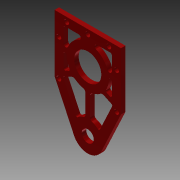
# Autodesk Inventor part: Swerve Wheel + Carriage Outline V1
Saved by Autodesk Inventor 2013 (Build 170138000, 138)
## iProperties
Created: 2013-04-01
Part Number: Swerve Wheel + Carriage Outline V1
Material: Generic
Document SubType Name: Sheet Metal
Designer: mvarma
Density: 1 g/cm^3
Sheet Metal Rule: Default
Author: mvarma
Autodesk Inventor part; units mm, degrees
ref_plane "YZ Plane" through (0, 0, 0) normal (1, 0, 0) x (0, 1, 0)
ref_plane "XZ Plane" through (0, 0, 0) normal (0, 1, 0) x (-1, 0, 0)
ref_plane "XY Plane" through (0, 0, 0) normal (0, 0, 1) x (1, 0, 0)
sketch "Sketch1" plane through (0, 0, 0) normal (0, 0, 1) x (1, 0, 0)
  circle A0 centre (0, 0) radius 38.1 construction
  circle A1 centre (0, 0) radius 41.275 construction
  line L0 (-7.332348, 0) -> (-3.666174, 6.35) construction
  line L1 (-3.666174, 6.35) -> (3.666174, 6.35) construction
  line L2 (3.666174, 6.35) -> (7.332348, 0) construction
  line L3 (7.332348, 0) -> (3.666174, -6.35) construction
  line L4 (3.666174, -6.35) -> (-3.666174, -6.35) construction
  line L5 (-3.666174, -6.35) -> (-7.332348, 0) construction
  circle A2 centre (0, 0) radius 6.35
  circle A3 centre (0, 0) radius 15.875 construction
  circle A4 centre (0, 0) radius 8.73125 construction
  arc A5 (0, 15.875) -> (-7.41955, 14.034454) centre (0, 0) ccw
  line L6 (34.925, 37.2364) -> (34.925, 97.5614)
  line L7 (34.925, 97.5614) -> (-34.925, 97.5614)
  line L8 (-34.925, 97.5614) -> (-34.925, 37.2364)
  line L9 (34.925, 37.2364) -> (-34.925, 37.2364) construction
  line L10 (34.925, 37.2364) -> (14.381959, -6.721227)
  line L11 (-34.925, 37.2364) -> (-14.381959, -6.721227)
  circle A6 centre (-30.353, 37.2364) radius 3.9624 construction
  line L12 (53.34, 97.5614) -> (-53.34, 97.5614) construction
  line L13 (-53.34, 97.5614) -> (-53.34, 107.0864) construction
  line L14 (-53.34, 107.0864) -> (53.34, 107.0864) construction
  line L15 (53.34, 107.0864) -> (53.34, 97.5614) construction
  circle A7 centre (-222.519943, 24.149358) radius 53.34 construction
  line L16 (-190.769943, 59.074358) -> (-254.269943, 59.074358) construction
  line L17 (-254.269943, 59.074358) -> (-254.269943, -10.775642) construction
  line L18 (-254.269943, -10.775642) -> (-190.769943, -10.775642) construction
  line L19 (-190.769943, -10.775642) -> (-190.769943, 59.074358) construction
  line L20 (-195.532443, 59.074358) -> (-195.532443, -10.775642) construction
  line L21 (-249.507443, 59.074358) -> (-249.507443, -10.775642) construction
  line L22 (-209.819943, 68.599358) -> (-235.219943, 68.599358) construction
  line L23 (-235.219943, 68.599358) -> (-235.219943, -20.300642) construction
  line L24 (-235.219943, -20.300642) -> (-209.819943, -20.300642) construction
  line L25 (-209.819943, -20.300642) -> (-209.819943, 68.599358) construction
  line L26 (34.925, 88.0364) -> (-34.925, 88.0364) construction
  circle A8 centre (30.353, 37.2364) radius 3.9624 construction
  circle A9 centre (30.353, 75.3364) radius 3.9624 construction
  circle A10 centre (-30.353, 75.3364) radius 3.9624 construction
  line L27 (34.925, 92.7989) -> (-34.925, 92.7989) construction
  circle A11 centre (0, 63.033275) radius 14.2875
  circle A12 centre (0, 63.033275) radius 15.875 construction
  line L28 (5.499261, 63.033275) -> (2.749631, 58.270775) construction
  line L29 (2.749631, 58.270775) -> (-2.749631, 58.270775) construction
  line L30 (-2.749631, 58.270775) -> (-5.499261, 63.033275) construction
  line L31 (-5.499261, 63.033275) -> (-2.749631, 67.795775) construction
  line L32 (-2.749631, 67.795775) -> (2.749631, 67.795775) construction
  line L33 (2.749631, 67.795775) -> (5.499261, 63.033275) construction
  line L34 (-34.925, 86.052025) -> (34.925, 86.052025) construction
  line L35 (34.925, 72.202675) -> (-34.925, 72.202675) construction
  line L36 (34.925, 89.6239) -> (-34.925, 89.6239) construction
  circle A13 centre (0, 0) radius 30.55 construction
  circle A14 centre (0, 63.033275) radius 11.45 construction
  line L37 (10.911689, 66.502792) -> (29.11372, 9.257095) construction
  line L38 (-10.911689, 66.502792) -> (-29.11372, 9.257095) construction
  line L39 (-10.911689, 66.502792) -> (0, 63.033275) construction
  line L40 (0, 63.033275) -> (10.911689, 66.502792) construction
  line L41 (0, 63.033275) -> (0, 0) construction
  line L42 (-23.495, 45.362532) -> (-23.495, 37.2364)
  circle A15 centre (0, 0) radius 15.875
  arc A16 (-7.41955, 14.034454) -> (8.47128, 13.425835) centre (0, 0) ccw
  circle A17 centre (0, 63.033275) radius 13.1318 construction
  point P0 (22.225, 92.7989)
  point P1 (0, 92.7989)
  point P2 (-22.225, 92.7989)
  dimension "d0" = 76.2
  dimension "d2" = 82.55
  dimension "d3" = 12.7
  dimension "d4" = 12.7
  dimension "d5" = 31.75
  dimension "d6" = 17.4625
  dimension "d8" = 69.85
  dimension "d9" = 34.925
  dimension "d10" = 37.2364
  dimension "d13" = 7.9248
  dimension "d14" = 9.525
  dimension "d15" = 106.68
  dimension "d16" = 53.34
  dimension "d17" = 106.68
  dimension "d18" = 69.85
  dimension "d19" = 34.925
  dimension "d20" = 63.5
  dimension "d21" = 31.75
  dimension "d22" = 4.7625
  dimension "d23" = 4.7625
  dimension "d24" = 25.4
  dimension "d25" = 14.2875
  dimension "d26" = 88.9
  dimension "d27" = 14.2875
  dimension "d28" = 44.45
  dimension "d29" = 4.572
  dimension "d30" = 9.525
  dimension "d31" = 0
  dimension "d32" = 7.9248
  dimension "d33" = 4.572
  dimension "d34" = 7.9248
  dimension "d35" = 7.9248
  dimension "d36" = 4.572
  dimension "d37" = 4.572
  dimension "d38" = 38.1
  dimension "d39" = 38.1
  dimension "d44" = 4.7625
  dimension "d45" = 34.925
  dimension "d46" = 12.7
  dimension "d47" = 12.7
  dimension "d48" = 28.575
  dimension "d52" = 31.75
  dimension "d53" = 9.525
  dimension "d54" = 25.00313
  dimension "d66" = 1.98438
  dimension "d67" = 9.1694
  dimension "d68" = 63.03327
  dimension "d69" = 13.84935
  dimension "d70" = 34.925
  dimension "d71" = 1.5875
  dimension "d74" = 144.722
  dimension "d75" = 60.06982
  dimension "d76" = 22.9
  dimension "d77" = 61.1
  dimension "d80" = 11.43
  dimension "d84" = 31.75
  dimension "d112" = 50.8
  dimension "d113" = 26.2636
  constraints: 86 end point, 20 point on line, 18 centre point, 17 point on circle, 16 coincident, 15 perpendicular, 8 tangent, 7 parallel, 5 horizontal, 1 midpoint, 27 other
  measures "d0" diameter of A0
  measures "d2" diameter of A1
  measures "d3" distance between parallel lines of L4 L1
  measures "d4" diameter of A2
  measures "d5" diameter of A3
  measures "d6" diameter of A4
  measures "d8" distance between parallel lines of L8 L6
  measures "d9" distance from line of point (0, 0) L8
  measures "d10" distance from line of L9 point (0, 0)
  measures "d13" diameter of A6
  measures "d14" distance of L14.end L12.start
  measures "d15" distance of L13.end L14.end
  measures "d16" horizontal distance of L12.start point (0, 0)
  measures "d17" diameter of A7
  measures "d18" distance of L18.end L16.start
  measures "d19" distance from line of A7.centre L18
  measures "d20" distance of L17.end L18.end
  measures "d21" distance from line of L19 A7.centre
  measures "d22" distance between parallel lines of L17 L21
  measures "d23" distance between parallel lines of L19 L20
  measures "d24" distance between parallel lines of L23 L25
  measures "d25" distance between parallel lines of L20 L25
  measures "d26" distance of L22.end L23.end
  measures "d27" distance between parallel lines of L21 L23
  measures "d28" distance from line of A7.centre L24
  measures "d29" distance from line of L8 A6.centre
  measures "d30" distance between parallel lines of L7 L26
  measures "d31" distance between parallel lines of L7 L12
  measures "d32" diameter of A8
  measures "d33" distance from line of L6 A8.centre
  measures "d34" diameter of A9
  measures "d35" diameter of A10
  measures "d36" distance from line of L8 A10.centre
  measures "d37" distance from line of L6 A9.centre
  measures "d38" distance from line of L9 A10.centre
  measures "d39" distance from line of L9 A9.centre
  measures "d44" distance between parallel lines of L26 L27
  measures "d45" distance from line of L8 point (0, 92.799)
  measures "d46" distance from line of L8 point (-22.225, 92.799)
  measures "d47" distance from line of L6 point (22.225, 92.799)
  measures "d48" diameter of A11
  measures "d52" diameter of A12
  measures "d53" distance between parallel lines of L29 L32
  measures "d54" distance from line of L26 A12.centre
  measures "d66" distance between parallel lines of L26 L34
  measures "d67" distance from line of L35 A11.centre
  measures "d68" distance of point (0, 0) A11.centre
  measures "d69" distance between parallel lines of L34 L35
  measures "d70" distance from line of L8 point (0, 63.033)
  measures "d71" distance between parallel lines of L26 L36
  measures "d74" angle of L40 L39
  measures "d75" distance of L37.start L37.end
  measures "d76" diameter of A14
  measures "d77" diameter of A13
  measures "d80" distance from line of L8 L42.end
  measures "d84" diameter of A15
  measures "d112" distance between parallel lines of L9 L26
  measures "d113" diameter of A17
extrude "Plate1" add sketch "Sketch1" along normal blind 4.7625 contours A2 | A15 A5 | A5 A15 L11 L8 L7 L6 L10 | A11
extrude "Cut1" cut sketch "Sketch1" along normal up to next contours A2 | A11
hole "Hole1" at (22.225, 92.7989, 0) at (0, 92.7989, 0) at (-22.225, 92.7989, 0) at (30.353, 75.3364, 0) at (30.353, 37.2364, 0) at (-30.353, 37.2364, 0) at (-30.353, 75.3364, 0) direction (0, 0, 1) diameter 4.9784 end through all clearance for "Socket Head Cap Screw" size "#10" standard "Ansi Unified Screw Threads"
sketch "Sketch2" plane through (0, 0, 0) normal (0, 0, -1) x (-1, 0, 0)
  circle A0 centre (0, 0) radius 6.35
  circle A1 centre (0, 63.033275) radius 14.2875
  arc A2 (-14.381959, -6.721227) -> (14.381959, -6.721227) centre (0, 0) ccw
  line L0 (34.925, 37.2364) -> (14.381959, -6.721227)
  line L1 (34.925, 97.5614) -> (34.925, 37.2364)
  line L2 (-34.925, 97.5614) -> (34.925, 97.5614)
  line L3 (-34.925, 37.2364) -> (-34.925, 97.5614)
  line L4 (-14.381959, -6.721227) -> (-34.925, 37.2364)
  line L5 (-24.857629, 41.941259) -> (-16.76236, 45.72448)
  line L6 (0, -15.875) -> (0, 97.5614)
  line L7 (24.857629, 41.941259) -> (16.76236, 45.72448)
  line L8 (-25.623702, 39.83094) -> (-12.865861, 12.531944)
  line L9 (12.865861, 12.531944) -> (25.623702, 39.83094)
  line L10 (0, -15.875) -> (0, -14.998192)
  arc A3 (-4.630208, 15.184755) -> (-10.388787, 12.003697) centre (0, 0) ccw
  arc A4 (4.861719, 41.346544) -> (13.49085, 45.371237) centre (0, 63.033275) ccw
  arc A5 (-24.857629, 41.941259) -> (-25.623702, 39.83094) centre (-24.185506, 40.503063) ccw
  arc A6 (25.623702, 39.83094) -> (24.857629, 41.941259) centre (24.185506, 40.503063) ccw
  arc A7 (10.388787, 12.003697) -> (4.630208, 15.184755) centre (0, 0) ccw
  arc A8 (-12.865861, 12.531944) -> (-10.388787, 12.003697) centre (-11.427665, 13.204066) ccw
  arc A9 (10.388787, 12.003697) -> (12.865861, 12.531944) centre (11.427665, 13.204066) ccw
  arc A10 (-13.49085, 45.371237) -> (-4.861719, 41.346544) centre (0, 63.033275) ccw
  arc A11 (19.163161, 51.776105) -> (22.223974, 62.8197) centre (0, 63.033275) ccw
  arc A12 (-13.49085, 45.371237) -> (-16.76236, 45.72448) centre (-15.418114, 42.848089) ccw
  arc A13 (16.76236, 45.72448) -> (13.49085, 45.371237) centre (15.418114, 42.848089) ccw
  line L11 (-25.623702, 39.83094) -> (-26.295825, 41.269136) construction
  line L12 (-24.857629, 41.941259) -> (-26.295825, 41.269136) construction
  line L13 (-23.140377, 48.000706) -> (-19.859836, 49.533826)
  line L14 (19.859836, 49.533826) -> (23.140377, 48.000706)
  line L15 (-25.4, 49.438902) -> (-25.4, 62.8197)
  line L16 (25.4, 49.438902) -> (25.4, 62.8197)
  line L17 (-25.4, 62.8197) -> (-22.223974, 62.8197) construction
  line L18 (25.4, 62.8197) -> (22.223974, 62.8197) construction
  arc A14 (-22.223974, 62.8197) -> (-25.4, 62.8197) centre (-23.811987, 62.8197) ccw
  arc A15 (25.4, 62.8197) -> (22.223974, 62.8197) centre (23.811987, 62.8197) ccw
  arc A16 (-25.4, 49.438902) -> (-23.140377, 48.000706) centre (-23.8125, 49.438902) ccw
  arc A17 (-19.859836, 49.533826) -> (-19.163161, 51.776105) centre (-20.531959, 50.972022) ccw
  arc A18 (19.163161, 51.776105) -> (19.859836, 49.533826) centre (20.531959, 50.972022) ccw
  arc A19 (23.140377, 48.000706) -> (25.4, 49.438902) centre (23.8125, 49.438902) ccw
  arc A20 (-22.223974, 62.8197) -> (-19.163161, 51.776105) centre (0, 63.033275) ccw
  arc A21 (22.223974, 62.8197) -> (20.791129, 70.88691) centre (0, 63.033275) ccw
  line L19 (-25.4, 62.8197) -> (-25.4, 86.4489)
  line L20 (-23.8125, 88.0364) -> (23.8125, 88.0364)
  line L21 (25.4, 86.4489) -> (25.4, 62.8197)
  arc A22 (-25.4, 71.728371) -> (-20.791129, 70.88691) centre (-23.01875, 71.728371) ccw
  arc A23 (-8.743968, 83.465936) -> (-9.680822, 88.0364) centre (-9.680822, 85.65515) ccw
  arc A24 (9.680822, 88.0364) -> (8.743968, 83.465936) centre (9.680822, 85.65515) ccw
  arc A25 (20.791129, 70.88691) -> (25.4, 71.728371) centre (23.01875, 71.728371) ccw
  arc A26 (-9.680822, 88.0364) -> (-8.743968, 83.465936) centre (-9.680822, 85.65515) ccw
  arc A27 (-20.791129, 70.88691) -> (-25.4, 71.728371) centre (-23.01875, 71.728371) ccw
  arc A28 (8.743968, 83.465936) -> (9.680822, 88.0364) centre (9.680822, 85.65515) ccw
  arc A29 (25.4, 71.728371) -> (20.791129, 70.88691) centre (23.01875, 71.728371) ccw
  arc A30 (20.791129, 70.88691) -> (8.743968, 83.465936) centre (0, 63.033275) ccw
  arc A31 (8.743968, 83.465936) -> (-8.743968, 83.465936) centre (0, 63.033275) ccw
  arc A32 (-8.743968, 83.465936) -> (-20.791129, 70.88691) centre (0, 63.033275) ccw
  arc A33 (-20.791129, 70.88691) -> (-22.223974, 62.8197) centre (0, 63.033275) ccw
  arc A34 (-23.8125, 88.0364) -> (-25.4, 86.4489) centre (-23.8125, 86.4489) ccw
  arc A35 (25.4, 86.4489) -> (23.8125, 88.0364) centre (23.8125, 86.4489) ccw
  line L22 (-2.38125, 38.248439) -> (-2.38125, 18.221706)
  line L23 (2.38125, 38.248439) -> (2.38125, 18.221706)
  arc A36 (-2.38125, 38.248439) -> (-4.861719, 41.346544) centre (-5.55625, 38.248439) ccw
  arc A37 (4.861719, 41.346544) -> (2.38125, 38.248439) centre (5.55625, 38.248439) ccw
  arc A38 (-4.630208, 15.184755) -> (-2.38125, 18.221706) centre (-5.55625, 18.221706) ccw
  arc A39 (2.38125, 18.221706) -> (4.630208, 15.184755) centre (5.55625, 18.221706) ccw
  point P0 (-34.925, 88.0364)
  point P1 (11.912889, 10.492792)
  point P2 (34.925, 88.0364)
  point P3 (-25.4, 46.9447)
  point P4 (25.4, 46.9447)
  point P5 (-2.38125, 40.93621)
  point P6 (-2.38125, 15.69539)
  point P7 (2.38125, 40.93621)
  point P8 (2.38125, 15.69539)
  dimension "d85" = 9.525
  dimension "d86" = 12.7
  dimension "d87" = 31.75
  dimension "d88" = 28.575
  dimension "d89" = 44.45
  dimension "d93" = 1.5875
  dimension "d94" = 1.5875
  dimension "d95" = 3.175
  dimension "d100" = 9.525
  dimension "d101" = 9.525
  dimension "d102" = 4.7625
  dimension "d103" = 15.875
  dimension "d104" = 15.875
  dimension "d105" = 1.5875
  dimension "d106" = 22.225
  dimension "d107" = 4.7625
  dimension "d108" = 9.525
  dimension "d109" = 4.7625
  dimension "d110" = 1.5875
  dimension "d114" = 4.7625
  dimension "d115" = 2.38125
  dimension "d116" = 3.175
  dimension "d117" = 22.225
  dimension "d118" = 3.175
  constraints: 88 point on circle, 43 tangent, 38 end point, 37 centre point, 19 point on line, 12 equal radius, 9 perpendicular, 5 parallel, 3 midpoint, 2 coincident, 2 collinear, 1 vertical
  measures "d85" distance between parallel lines of L0 L9
  measures "d86" diameter of A0
  measures "d87" diameter of A3
  measures "d88" diameter of A1
  measures "d89" diameter of A4
  measures "d93" radius of A5
  measures "d94" radius of A8
  measures "d95" radius of A12
  measures "d100" distance between parallel lines of L3 L15
  measures "d101" distance between parallel lines of L1 L16
  measures "d102" distance between parallel lines of L13 L5
  measures "d103" distance of point (-25.4, 46.945) L15.end
  measures "d104" distance of point (25.4, 46.945) L16.end
  measures "d105" radius of A16
  measures "d106" radius of A11
  measures "d107" distance between parallel lines of L7 L14
  measures "d108" distance between parallel lines of L2 L20
  measures "d109" diameter of A25
  measures "d110" radius of A34
  measures "d114" distance between parallel lines of L23 L22
  measures "d115" distance between parallel lines of L6 L23
  measures "d116" radius of A36
  measures "d117" radius of A10
  measures "d118" radius of A38
sketch "Sketch2 outline for Cut2" plane through (0, 0, 0) normal (0, 0, -1) x (-1, 0, 0)
  line L0 (25.623702, 39.83094) -> (12.865861, 12.531944)
  arc A0 (12.865861, 12.531944) -> (10.388787, 12.003697) centre (11.427665, 13.204066) cw
  arc A1 (10.388787, 12.003697) -> (4.630208, 15.184755) centre (0, 0) ccw
  arc A2 (4.630208, 15.184755) -> (2.38125, 18.221706) centre (5.55625, 18.221706) cw
  line L1 (2.38125, 18.221706) -> (2.38125, 38.248439)
  arc A3 (2.38125, 38.248439) -> (4.861719, 41.346544) centre (5.55625, 38.248439) cw
  arc A4 (4.861719, 41.346544) -> (13.49085, 45.371237) centre (0, 63.033275) ccw
  arc A5 (13.49085, 45.371237) -> (16.76236, 45.72448) centre (15.418114, 42.848089) cw
  line L2 (16.76236, 45.72448) -> (24.857629, 41.941259)
  arc A6 (24.857629, 41.941259) -> (25.623702, 39.83094) centre (24.185506, 40.503063) cw
  arc A7 (-24.857629, 41.941259) -> (-25.623702, 39.83094) centre (-24.185506, 40.503063) ccw
  line L3 (-16.76236, 45.72448) -> (-24.857629, 41.941259)
  arc A8 (-13.49085, 45.371237) -> (-16.76236, 45.72448) centre (-15.418114, 42.848089) ccw
  arc A9 (-4.861719, 41.346544) -> (-13.49085, 45.371237) centre (0, 63.033275) cw
  arc A10 (-2.38125, 38.248439) -> (-4.861719, 41.346544) centre (-5.55625, 38.248439) ccw
  line L4 (-2.38125, 18.221706) -> (-2.38125, 38.248439)
  arc A11 (-4.630208, 15.184755) -> (-2.38125, 18.221706) centre (-5.55625, 18.221706) ccw
  arc A12 (-10.388787, 12.003697) -> (-4.630208, 15.184755) centre (0, 0) cw
  arc A13 (-12.865861, 12.531944) -> (-10.388787, 12.003697) centre (-11.427665, 13.204066) ccw
  line L5 (-25.623702, 39.83094) -> (-12.865861, 12.531944)
  arc A14 (20.791129, 70.88691) -> (25.4, 71.728371) centre (23.01875, 71.728371) ccw
  line L6 (25.4, 71.728371) -> (25.4, 86.4489)
  arc A15 (25.4, 86.4489) -> (23.8125, 88.0364) centre (23.8125, 86.4489) ccw
  line L7 (23.8125, 88.0364) -> (9.680822, 88.0364)
  arc A16 (9.680822, 88.0364) -> (8.743968, 83.465936) centre (9.680822, 85.65515) ccw
  arc A17 (8.743968, 83.465936) -> (20.791129, 70.88691) centre (0, 63.033275) cw
  line L8 (25.4, 49.438902) -> (25.4, 62.8197)
  arc A18 (23.140377, 48.000706) -> (25.4, 49.438902) centre (23.8125, 49.438902) ccw
  line L9 (19.859836, 49.533826) -> (23.140377, 48.000706)
  arc A19 (19.163161, 51.776105) -> (19.859836, 49.533826) centre (20.531959, 50.972022) ccw
  arc A20 (22.223974, 62.8197) -> (19.163161, 51.776105) centre (0, 63.033275) cw
  arc A21 (25.4, 62.8197) -> (22.223974, 62.8197) centre (23.811987, 62.8197) ccw
  arc A22 (-8.743968, 83.465936) -> (-9.680822, 88.0364) centre (-9.680822, 85.65515) ccw
  line L10 (-9.680822, 88.0364) -> (-23.8125, 88.0364)
  arc A23 (-23.8125, 88.0364) -> (-25.4, 86.4489) centre (-23.8125, 86.4489) ccw
  line L11 (-25.4, 86.4489) -> (-25.4, 71.728371)
  arc A24 (-25.4, 71.728371) -> (-20.791129, 70.88691) centre (-23.01875, 71.728371) ccw
  arc A25 (-20.791129, 70.88691) -> (-8.743968, 83.465936) centre (0, 63.033275) cw
  arc A26 (-22.223974, 62.8197) -> (-25.4, 62.8197) centre (-23.811987, 62.8197) ccw
  arc A27 (-19.163161, 51.776105) -> (-22.223974, 62.8197) centre (0, 63.033275) cw
  arc A28 (-19.859836, 49.533826) -> (-19.163161, 51.776105) centre (-20.531959, 50.972022) ccw
  line L12 (-23.140377, 48.000706) -> (-19.859836, 49.533826)
  arc A29 (-25.4, 49.438902) -> (-23.140377, 48.000706) centre (-23.8125, 49.438902) ccw
  line L13 (-25.4, 62.8197) -> (-25.4, 49.438902)
extrude "Cut2" cut sketch "Sketch2 outline for Cut2" against normal blind 4.7625
equation "\"d16\" = 0.5 * d15"
equation "\"d45\" = d42"
equation "\"d47\" = d46"
equation "\"d56\" = Thickness"
equation "\"d19\" = 0.5 * d18"
equation "\"d21\" = 0.5 * d20"
equation "\"d22\" = d23"
equation "\"d25\" = d27"
equation "\"d28\" = 0.5 * d26"
equation "\"d32\" = d13"
equation "\"d33\" = d29"
equation "\"d34\" = d32"
equation "\"d35\" = d13"
equation "\"d36\" = d29"
equation "\"d37\" = d29"
equation "\"d39\" = d38"
equation "\"d44\" = 0.5 * d30"
equation "\"d63\" = Thickness"
equation "\"BendRadius\" = Thickness"
equation "\"BendReliefWidth\" = Thickness"
equation "\"BendReliefDepth\" = 0.5 * Thickness"
equation "\"CornerReliefSize\" = 4 * Thickness"
equation "\"MinimumRemnant\" = 2 * Thickness"
equation "\"TransitionRadius\" = BendRadius"
equation "\"JacobiRadiusSize\" = Thickness"
equation "\"GapSize\" = Thickness"
equation "\"d55\" = BendRadius"
equation "\"Thickness\" = 4.7625"
equation "\"d42\" = 34.925"
body "Solid1"
